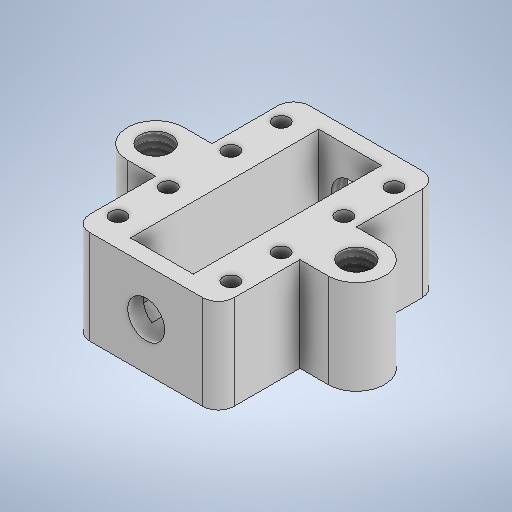
# Autodesk Inventor part: 15
Saved by Autodesk Inventor 2025.1 (Build 291241000, 241)
## iProperties
Created: 2024-09-13
Part Number: 15
Material: Generisch
Document SubType Name: Modeling
Designer: ffogue
Density: 1 g/cm^3
Appearance: Vorgabe
Author: ffogue
Autodesk Inventor part; units mm, degrees
note: some values were not read from the file. Chosen so that the rebuilt part matches the saved one: direction of "Hole1"; direction of "Hole3".
ref_plane "YZ Plane" through (0, 0, 0) normal (1, 0, 0) x (0, 1, 0)
ref_plane "XZ Plane" through (0, 0, 0) normal (0, 1, 0) x (-1, 0, 0)
ref_plane "XY Plane" through (0, 0, 0) normal (0, 0, 1) x (1, 0, 0)
sketch "Sketch1" plane through (0, 0, 0) normal (0, 0, 1) x (1, 0, 0)
  line L0 (-11.5, -17.5) -> (11.5, -17.5)
  line L1 (11.5, -17.5) -> (11.5, 17.5)
  line L2 (11.5, 17.5) -> (-11.5, 17.5)
  line L3 (-11.5, 17.5) -> (-11.5, -17.5)
  line L4 (-11.5, -17.5) -> (11.5, 17.5) construction
  line L5 (11.5, -17.5) -> (-11.5, 17.5) construction
  line L6 (-11.5, 4.5) -> (-16, 4.5)
  line L7 (-20.5, 0) -> (-20.5, 0)
  line L8 (-16, -4.5) -> (-11.5, -4.5)
  line L9 (11.5, 4.5) -> (16, 4.5)
  line L10 (20.5, 0) -> (20.5, 0)
  line L11 (16, -4.5) -> (11.5, -4.5)
  arc A0 (16, -4.5) -> (20.5, 0) centre (16, 0) ccw
  arc A1 (20.5, 0) -> (16, 4.5) centre (16, 0) ccw
  arc A2 (-20.5, 0) -> (-16, -4.5) centre (-16, 0) ccw
  arc A3 (-16, 4.5) -> (-20.5, 0) centre (-16, 0) ccw
  point P0 (0, 0)
  point P1 (-20.5, 0)
  point P2 (-11.5, 0)
  point P3 (20.5, 0)
  point P4 (11.5, 0)
  point P5 (13.75, -4.5)
  point P6 (0, -17.5)
  point P7 (20.5, 0)
  dimension "d0" = 35
  dimension "d1" = 23
  dimension "d2" = 4.5
  dimension "d3" = 9
  dimension "d4" = 4.5
  dimension "d5" = 9
  dimension "d6" = 32
  dimension "d7" = 16
  constraints: 24 end point, 8 midpoint, 8 point on circle, 8 tangent, 6 perpendicular, 4 centre point, 4 point on line, 2 equal radius, 2 horizontal, 2 horizontal alignment, 2 parallel
  measures "d0" distance of L0.end L1.end
  measures "d1" distance of L1.end L2.end
  measures "d2" radius of A0
  measures "d3" distance from line of point (13.75, -4.5) L9
  measures "d4" radius of A3
  measures "d5" distance between parallel lines of L8 L6
  measures "d6" distance of A0.centre A2.centre
  measures "d7" horizontal distance of point (0, -17.5) A2.centre
extrude "Extrusion1" add sketch "Sketch1" along normal mid plane 15
sketch "Sketch2" plane through (0, 0, 7.5) normal (0, 0, 1) x (1, 0, 0)
  arc A0 (-16, 4.5) -> (-16, -4.5) centre (-16, 0) ccw projected
  arc A1 (16, -4.5) -> (16, 4.5) centre (16, 0) ccw projected
  point P0 (0, 0)
  point P1 (-16, 0)
  point P2 (16, 0)
  constraints: 2 coincident
hole "Hole1" at (-16, 0, 7.5) at (16, 0, 7.5) direction (0, 0, -1) diameter 4.917 depth 15 thread size "M6x1" class "6H" standard "ISO Metric profile"
sketch "Sketch4" plane through (-11.5, 17.5, 7.5) normal (0, 1, 0) x (1, 0, 0)
  point P0 (11.5, 7.5)
  point P1 (11.5, 7.5)
  constraints: 1 coincident
hole "Hole2" at (0, 17.5, 0) direction (0, -1, 0) diameter 5.9175 end through all thread size "M7x1" class "6H" standard "ISO Metric profile"
sketch "Sketch3" plane through (0, 0, 7.5) normal (0, 0, 1) x (1, 0, 0)
  line L0 (-5, -15) -> (5, -15)
  line L1 (5, -15) -> (5, 15)
  line L2 (5, 15) -> (-5, 15)
  line L3 (-5, 15) -> (-5, -15)
  line L4 (-5, -15) -> (5, 15) construction
  line L5 (5, -15) -> (-5, 15) construction
  point P0 (0, 0)
  dimension "d17" = 10
  dimension "d18" = 30
  constraints: 12 end point, 2 midpoint, 2 parallel, 1 horizontal, 1 perpendicular
  measures "d17" distance of L1.end L2.end
  measures "d18" distance of L0.end L1.end
extrude "Extrusion2" cut sketch "Sketch3" against normal blind 10
sketch "Sketch6" plane through (0, 0, 7.5) normal (0, 0, 1) x (1, 0, 0)
  line L0 (-11.5, -17.5) -> (11.5, -17.5) projected
  point P0 (0, 0)
  point P1 (-9, -13)
  point P2 (-9, -5)
  point P3 (9, -5)
  point P4 (9, -13)
  dimension "d31" = 8
  dimension "d42" = 5
  dimension "d43" = 18
  dimension "d44" = 9
  constraints: 2 horizontal alignment, 2 vertical alignment
  measures "d31" distance of point (9, -5) point (9, -13)
  measures "d42" vertical distance of point (0, 0) point (9, -5)
  measures "d43" distance of point (-9, -13) point (9, -13)
  measures "d44" horizontal distance of point (0, 0) point (9, -13)
hole "Hole3" at (-9, -13, 7.5) at (-9, -5, 7.5) at (9, -5, 7.5) at (9, -13, 7.5) direction (0, 0, -1) diameter 2.5 depth 15
mirror "Mirror1" about plane through (0, 0, 0) normal (0, 1, 0) of "Hole3"
fillet "Fillet1" radius 2.5 6 edges at (11.5, 17.5, 3.75) (11.5, 17.5, -3.75) (-11.5, 17.5, 3.75) (-11.5, 17.5, -3.75) (-11.5, -17.5, 0) (11.5, -17.5, 0)
equation "\"d5\" = d3"
equation "\"d7\" = 0.5 * d6"
body "Solid1"
